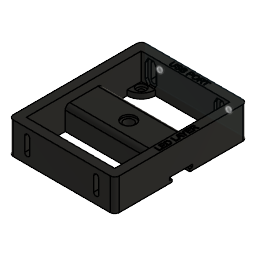
LED-LAYER (Autodesk Fusion 360 design; units mm, degrees)
part number: 2026-05-15-16-15-28-168
Autodesk Fusion 360 part; units mm, degrees
note: some values were not read from the file. Chosen so that the rebuilt part matches the saved one: which face or edge a step refers to; a direction; the layout of a text. Set by a fixed rule: which sketch regions a step uses.
sketch "Sketch1" plane through (0, 0, 0) normal (0, 0, 1) x (1, 0, 0)
  line L0 (2.5, 0) -> (57.5, 0)
  line L1 (60, 2.5) -> (60, 72.5)
  line L2 (57.5, 75) -> (2.5, 75)
  line L3 (0, 72.5) -> (0, 2.5)
  arc A0 (0, 2.5) -> (2.5, 0) centre (2.5, 2.5) ccw
  arc A1 (57.5, 0) -> (60, 2.5) centre (57.5, 2.5) ccw
  arc A2 (60, 72.5) -> (57.5, 75) centre (57.5, 72.5) ccw
  arc A3 (2.5, 75) -> (0, 72.5) centre (2.5, 72.5) ccw
  point P0 (60, 0)
  point P1 (0, 75)
  dimension "d1" = 60
  dimension "d2" = 75
  dimension "d3" = 2.5
  constraint horizontal L0
  constraint vertical L1
  constraint horizontal L2
  constraint vertical L3
  constraint coincident origin L0
  constraint coincident origin L3
  constraint tangent L0 A0
  constraint tangent L3 A0
  constraint coincident P0 L0
  constraint coincident P0 L1
  constraint tangent L0 A1
  constraint tangent L1 A1
  constraint equal A0 A1
  constraint tangent L1 A2
  constraint tangent L2 A2
  constraint equal A0 A2
  constraint coincident P1 L2
  constraint coincident P1 L3
  constraint tangent L2 A3
  constraint tangent L3 A3
  constraint equal A0 A3
  measures "d1" distance of origin P0
  measures "d2" distance of origin P1
  measures "d3" radius of A0
extrude "Extrude1" add sketch "Sketch1" along normal blind 6
sketch "Sketch2" plane through (60, 0, 0) normal (1, 0, 0) x (0, 1, 0)
  line L0 (2.5, 0) -> (72.5, 0)
  line L1 (72.5, 0) -> (72.5, 6)
  line L2 (72.5, 6) -> (2.5, 6)
  line L3 (2.5, 6) -> (2.5, 0)
  line L4 (32.5, 0) -> (42.5, 0)
  line L5 (42.5, 0) -> (42.5, 3)
  line L6 (42.5, 3) -> (32.5, 3)
  line L7 (32.5, 3) -> (32.5, 0)
  line L8 (0, 0) -> (0, 6)
  dimension "d6" = 10
  dimension "d7" = 3
  dimension "d8" = 32.5
  constraint horizontal L4
  constraint vertical L5
  constraint horizontal L6
  constraint vertical L7
  constraint coincident L0 L4.start
  measures "d6" distance of L4.start L4.end
  measures "d7" distance of L4.start L6.end
  measures "d8" distance of L7 L8
extrude "Extrude2" cut sketch "Sketch2" against normal blind 60 contours L0 L4 L5 L6 L7
sketch "Sketch3" plane through (60, 0, 0) normal (1, 0, 0) x (0, 1, 0)
  line L0 (42.5, 3) -> (42.5, 0)
  line L1 (42.5, 0) -> (72.5, 0)
  line L2 (72.5, 0) -> (72.5, 6)
  line L3 (72.5, 6) -> (2.5, 6)
  line L4 (2.5, 6) -> (2.5, 0)
  line L5 (2.5, 0) -> (32.5, 0)
  line L6 (32.5, 0) -> (32.5, 3)
  line L7 (32.5, 3) -> (42.5, 3)
  line L8 (30, 5) -> (45, 5)
  line L9 (45, 5) -> (45, 3)
  line L10 (45, 3) -> (30, 3)
  line L11 (30, 3) -> (30, 5)
  dimension "d11" = 2.5
  constraint horizontal L8
  constraint vertical L9
  constraint horizontal L10
  constraint vertical L11
  measures "d11" distance of L6 L11
extrude "Extrude3" cut sketch "Sketch3" along normal blind 60 contours L7 L8 L9 L10 L11
sketch "Sketch4" plane through (0, 0, 6) normal (0, 0, 1) x (-1, 0, 0)
  arc A0 (-2.5, -75) -> (0, -72.5) centre (-2.5, -72.5) ccw
  line L0 (0, -72.5) -> (0, -2.5)
  arc A1 (0, -2.5) -> (-2.5, 0) centre (-2.5, -2.5) ccw
  line L1 (-2.5, 0) -> (-57.5, 0)
  arc A2 (-57.5, 0) -> (-60, -2.5) centre (-57.5, -2.5) ccw
  line L2 (-60, -2.5) -> (-60, -72.5)
  arc A3 (-60, -72.5) -> (-57.5, -75) centre (-57.5, -72.5) ccw
  line L3 (-57.5, -75) -> (-2.5, -75)
  circle A4 centre (-29.575, -37.5) radius 2.6
  line L4 (-5, -5) -> (-55, -5)
  line L5 (-55, -5) -> (-55, -70)
  line L6 (-55, -70) -> (-5, -70)
  line L7 (-5, -70) -> (-5, -5)
  dimension "d14" = 5.2
  dimension "d15" = 37.5
  dimension "d16" = 30.425
  constraint horizontal L4
  constraint vertical L5
  constraint horizontal L6
  constraint vertical L7
  measures "d14" diameter of A4
  measures "d15" distance of L1 A4.centre
  measures "d16" distance of L2 A4.centre
extrude "Extrude4" add sketch "Sketch4" along normal blind 7 contours A0 L0 A1 L1 A2 L2 A3 L3 | L4 L5 L6 L7
extrude "Extrude5" cut 1 faces at (30.432, 36.8771, 6) along direction (0, 0, -1) blind 1
extrude "Extrude6" cut sketch "Sketch4" against normal blind 1 contours L4 L5 L6 L7
sketch "Sketch5" plane through (0, 0, 13) normal (0, 0, 1) x (-1, 0, 0)
  circle A0 centre (-29.575, -37.5) radius 2.6
  line L0 (-57.5, -75) -> (-2.5, -75)
  arc A1 (-2.5, -75) -> (0, -72.5) centre (-2.5, -72.5) ccw
  line L1 (0, -72.5) -> (0, -2.5)
  arc A2 (0, -2.5) -> (-2.5, 0) centre (-2.5, -2.5) ccw
  line L2 (-2.5, 0) -> (-57.5, 0)
  arc A3 (-57.5, 0) -> (-60, -2.5) centre (-57.5, -2.5) ccw
  line L3 (-60, -2.5) -> (-60, -72.5)
  arc A4 (-60, -72.5) -> (-57.5, -75) centre (-57.5, -72.5) ccw
  line L4 (-5, -5) -> (-55, -5)
  line L5 (-55, -5) -> (-55, -70)
  line L6 (-55, -70) -> (-5, -70)
  line L7 (-5, -70) -> (-5, -5)
  circle A5 centre (-29.575, -37.5) radius 5
  line L8 (-5, -30) -> (-55, -30)
  line L9 (-55, -30) -> (-55, -45)
  line L10 (-55, -45) -> (-5, -45)
  line L11 (-5, -45) -> (-5, -30)
  dimension "d23" = 10
  constraint horizontal L4
  constraint vertical L5
  constraint horizontal L6
  constraint vertical L7
  constraint concentric A0 A5
  constraint horizontal L8
  constraint vertical L9
  constraint horizontal L10
  constraint vertical L11
  constraint coincident L5 L9.end
  constraint coincident L7 L8.start
  measures "d23" diameter of A5
extrude "Extrude7" cut sketch "Sketch5" against normal blind 7 contours L4 L5 L7 L8 | L5 L6 L7 L10
sketch "Sketch6" plane through (0, 0, 13) normal (0, 0, 1) x (-1, 0, 0)
  line L0 (-5, -27) -> (-55, -27)
  line L1 (-55, -27) -> (-55, -5)
  line L2 (-55, -5) -> (-5, -5)
  line L3 (-5, -5) -> (-5, -27)
  line L4 (-5, -48) -> (-55, -48)
  line L5 (-55, -48) -> (-55, -70)
  line L6 (-55, -70) -> (-5, -70)
  line L7 (-5, -70) -> (-5, -48)
  constraint horizontal L0
  constraint vertical L1
  constraint horizontal L2
  constraint vertical L3
  constraint horizontal L4
  constraint vertical L5
  constraint horizontal L6
  constraint vertical L7
extrude "Extrude9" cut sketch "Sketch6" against normal blind 20
sketch "Sketch7" plane through (0, 0, 13) normal (0, 0, 1) x (-1, 0, 0)
  line L0 (-5, -45) -> (-5, -70)
  line L1 (-5, -70) -> (-55, -70)
  line L2 (-55, -70) -> (-55, -45)
  line L3 (-55, -45) -> (-5, -45)
  line L4 (-55, -30) -> (-55, -5)
  line L5 (-55, -5) -> (-5, -5)
  line L6 (-5, -5) -> (-5, -30)
  line L7 (-5, -30) -> (-55, -30)
  circle A0 centre (-29.575, -37.5) radius 2.6
  line L8 (-57.5, -75) -> (-2.5, -75)
  arc A1 (-2.5, -75) -> (0, -72.5) centre (-2.5, -72.5) ccw
  line L9 (0, -72.5) -> (0, -2.5)
  arc A2 (0, -2.5) -> (-2.5, 0) centre (-2.5, -2.5) ccw
  line L10 (-2.5, 0) -> (-57.5, 0)
  arc A3 (-57.5, 0) -> (-60, -2.5) centre (-57.5, -2.5) ccw
  line L11 (-60, -2.5) -> (-60, -72.5)
  arc A4 (-60, -72.5) -> (-57.5, -75) centre (-57.5, -72.5) ccw
  line L12 (-5, -30) -> (-5, -45)
  line L13 (-55, -45) -> (-55, -30)
  constraint coincident L6.end L7.start
  constraint coincident L0.start L3.end
  constraint coincident L2.end L3.start
  constraint coincident L4.start L7.end
extrude "Extrude10" add sketch "Sketch7" along normal blind 5 contours L8 A1 L9 A2 L10 A3 L11 A4
sketch "Sketch8" plane through (0, 5, 0) normal (0, 1, 0) x (-1, 0, 0)
  line L0 (-55, 13) -> (-55, 0)
  line L1 (-55, 0) -> (-5, 0)
  line L2 (-5, 0) -> (-5, 18)
  line L3 (-5, 18) -> (-55, 18)
  line L4 (-55, 18) -> (-55, 13)
  line L5 (-5, 0) -> (-13, 0)
  line L6 (-13, 0) -> (-13, 3)
  line L7 (-13, 3) -> (-5, 3)
  line L8 (-5, 3) -> (-5, 0)
  line L9 (-55, 0) -> (-47, 0)
  line L10 (-47, 0) -> (-47, 3)
  line L11 (-47, 3) -> (-55, 3)
  line L12 (-55, 3) -> (-55, 0)
  dimension "d32" = 8
  dimension "d33" = 3
  dimension "d34" = 8
  dimension "d35" = 3
  constraint horizontal L5
  constraint vertical L6
  constraint horizontal L7
  constraint vertical L8
  constraint coincident L1.end L2.start
  constraint horizontal L9
  constraint vertical L10
  constraint horizontal L11
  constraint vertical L12
  constraint coincident L0.end L1.start
  measures "d32" distance of L1.end L5.end
  measures "d33" distance of L1.end L7.end
  measures "d34" distance of L0.end L9.end
  measures "d35" distance of L0.end L11.end
extrude "Extrude11" add sketch "Sketch8" along normal blind 8 contours L0 L1 L9 L10 L11 L12 | L1 L2 L5 L6 L7 L8
sketch "Sketch9" plane through (0, 70, 0) normal (0, -1, 0) x (1, 0, 0)
  line L0 (5, 18) -> (5, 0)
  line L1 (5, 0) -> (55, 0)
  line L2 (55, 0) -> (55, 13)
  line L3 (55, 13) -> (55, 18)
  line L4 (55, 18) -> (5, 18)
  line L5 (5, 0) -> (13, 0)
  line L6 (13, 0) -> (13, 3)
  line L7 (13, 3) -> (5, 3)
  line L8 (5, 3) -> (5, 0)
  line L9 (55, 0) -> (47, 0)
  line L10 (47, 0) -> (47, 3)
  line L11 (47, 3) -> (55, 3)
  line L12 (55, 3) -> (55, 0)
  dimension "d38" = 8
  dimension "d39" = 3
  dimension "d40" = 8
  dimension "d41" = 3
  constraint horizontal L5
  constraint vertical L6
  constraint horizontal L7
  constraint vertical L8
  constraint coincident L0.end L1.start
  constraint horizontal L9
  constraint vertical L10
  constraint horizontal L11
  constraint vertical L12
  constraint coincident L1.end L2.start
  measures "d38" distance of L0.end L5.end
  measures "d39" distance of L0.end L7.end
  measures "d40" distance of L1.end L9.end
  measures "d41" distance of L1.end L11.end
extrude "Extrude12" add sketch "Sketch9" along normal blind 8 contours L0 L1 L5 L6 L7 L8 | L1 L2 L9 L10 L11 L12
extrude "Extrude13" add 2 faces at (21.6667, 41, 5) (21.6667, 41, 5) along direction (0, 0, 1) blind 8
sketch "Sketch10" plane through (0, 0, 3) normal (0, 0, 1) x (-1, 0, 0)
  line L0 (-55, -70) -> (-47, -70)
  line L1 (-47, -70) -> (-47, -62)
  line L2 (-47, -62) -> (-55, -62)
  line L3 (-55, -62) -> (-55, -70)
  circle A0 centre (-52, -67) radius 1.4
  line L4 (-55, -5) -> (-55, -70)
  line L5 (-55, -70) -> (-5, -70)
  circle A1 centre (-52, -8) radius 1.4
  line L6 (-5, -5) -> (-55, -5)
  circle A2 centre (-8, -67) radius 1.4
  line L7 (-5, -70) -> (-5, -5)
  circle A3 centre (-8, -8) radius 1.4
  dimension "d46" = 2.8
  dimension "d47" = 3
  dimension "d48" = 3
  dimension "d49" = 2.8
  dimension "d50" = 3
  dimension "d51" = 3
  dimension "d52" = 2.8
  dimension "d53" = 3
  dimension "d54" = 3
  dimension "d55" = 2.8
  dimension "d56" = 3
  dimension "d57" = 3
  measures "d46" diameter of A0
  measures "d47" distance of A0.centre L4
  measures "d48" distance of A0.centre L5
  measures "d49" diameter of A1
  measures "d50" distance of L4 A1.centre
  measures "d51" distance of A1.centre L6
  measures "d52" diameter of A2
  measures "d53" distance of L5 A2.centre
  measures "d54" distance of A2.centre L7
  measures "d55" diameter of A3
  measures "d56" distance of L6 A3.centre
  measures "d57" distance of L7 A3.centre
extrude "Extrude14" cut sketch "Sketch10" against normal blind 3 contours A0 | A1 | A2 | A3
sketch "Sketch11" plane through (0, 0, 3) normal (0, 0, 1) x (-1, 0, 0)
  circle A0 centre (-52, -67) radius 1.4
  line L0 (-55, -70) -> (-47, -70)
  line L1 (-47, -70) -> (-47, -62)
  line L2 (-47, -62) -> (-55, -62)
  line L3 (-55, -62) -> (-55, -70)
  arc A1 (-47, -70) -> (-55, -62) centre (-55, -70) ccw
  arc A2 (-5, -62) -> (-13, -70) centre (-5, -70) ccw
  arc A3 (-13, -5) -> (-5, -13) centre (-5, -5) ccw
  arc A4 (-55, -13) -> (-47, -5) centre (-55, -5) ccw
  line L4 (-13, -70) -> (-13, -62)
  line L5 (-13, -62) -> (-5, -62)
  line L6 (-5, -13) -> (-13, -13)
  line L7 (-13, -13) -> (-13, -5)
  line L8 (-55, -13) -> (-47, -13)
  line L9 (-47, -13) -> (-47, -5)
  constraint coincident L0 L1.start
  constraint coincident L2.end L3.start
  constraint coincident L0.start L3.end
  constraint tangent A2 L4
  constraint vertical L4
  constraint tangent A2 L5
  constraint tangent A3 L6
  constraint parallel L5 L6
  constraint tangent A3 L7
  constraint tangent A4 L8
  constraint perpendicular L7 L8
  constraint tangent A4 L9
extrude "Extrude15" cut sketch "Sketch11" against normal blind 3 contours L1 L2 A1 | A2 L4 L5 | A3 L6 L7 | A4 L8 L9
sketch "Sketch12" plane through (0, 0, 18) normal (0, 0, 1) x (-1, 0, 0)
  line L0 (-55, -70) -> (-55, -45)
  line L1 (-55, -45) -> (-55, -30)
  line L2 (-55, -30) -> (-55, -5)
  line L3 (-55, -5) -> (-5, -5)
  line L4 (-5, -5) -> (-5, -70)
  line L5 (-5, -70) -> (-55, -70)
  arc A0 (-60, -72.5) -> (-57.5, -75) centre (-57.5, -72.5) ccw
  line L6 (-57.5, -75) -> (-2.5, -75)
  arc A1 (-2.5, -75) -> (0, -72.5) centre (-2.5, -72.5) ccw
  line L7 (0, -72.5) -> (0, -2.5)
  arc A2 (0, -2.5) -> (-2.5, 0) centre (-2.5, -2.5) ccw
  line L8 (-2.5, 0) -> (-57.5, 0)
  arc A3 (-57.5, 0) -> (-60, -2.5) centre (-57.5, -2.5) ccw
  line L9 (-60, -2.5) -> (-60, -72.5)
  line L10 (-13, -70) -> (-47, -70) construction
  line L11 (-47, -70) -> (-47, -75) construction
  line L12 (-47, -75) -> (-13, -75) construction
  line L13 (-13, -75) -> (-13, -70) construction
  line L14 (-60, -13) -> (-60, -62) construction
  line L15 (-60, -62) -> (-55, -62) construction
  line L16 (-55, -62) -> (-55, -13) construction
  line L17 (-55, -13) -> (-60, -13) construction
  dimension "d62" = 3
  dimension "d64" = 3
  text T0 "USB PORT" font "Arial" height 3 align centre middle in box 34 x 5 at (-13, -70) x (-1, 0) y (0, -1) spacing 1 kerned
  text T1 "LED LAYER" font "Arial" height 3 align centre middle in box 49 x 5 at (-60, -13) x (0, -1) y (1, 0) spacing 1 kerned
  constraint coincident L6
  constraint coincident L5
  constraint coincident L0
  constraint coincident L9
extrude "Extrude16" cut sketch "Sketch12" against normal blind 2 text T1 T0
fillet "Fillet1" radius 2.5 2 edges at (30, 48, 13) (30, 27, 13)
sketch "Sketch13" plane through (0, 0, 0) normal (0, -1, 0) x (1, 0, 0)
  line L0 (2.5, 0) -> (57.5, 0)
  line L1 (57.5, 0) -> (57.5, 18)
  line L2 (57.5, 18) -> (2.5, 18)
  line L3 (2.5, 18) -> (2.5, 0)
  circle A0 centre (10.5, 9) radius 1.4
  circle A1 centre (49.5, 9) radius 1.4
  dimension "d70" = 2.8
  dimension "d71" = 9
  dimension "d72" = 8
  dimension "d73" = 2.8
  dimension "d74" = 8
  dimension "d75" = 9
  measures "d70" diameter of A0
  measures "d71" distance of L2 A0.centre
  measures "d72" distance of L3 A0.centre
  measures "d73" diameter of A1
  measures "d74" distance of L1 A1.centre
  measures "d75" distance of L2 A1.centre
extrude "Extrude17" cut sketch "Sketch13" against normal blind 6 contours A0 | A1
sketch "Sketch14" plane through (0, 75, 0) normal (0, 1, 0) x (-1, 0, 0)
  line L0 (-57.5, 0) -> (-2.5, 0)
  line L1 (-2.5, 0) -> (-2.5, 18)
  line L2 (-2.5, 18) -> (-57.5, 18)
  line L3 (-57.5, 18) -> (-57.5, 0)
  circle A0 centre (-49.5, 9) radius 1.4
  circle A1 centre (-10.5, 9) radius 1.4
  dimension "d78" = 2.8
  dimension "d79" = 9
  dimension "d80" = 8
  dimension "d81" = 2.8
  dimension "d82" = 9
  dimension "d83" = 8
  measures "d78" diameter of A0
  measures "d79" distance of L0 A0.centre
  measures "d80" distance of L3 A0.centre
  measures "d81" diameter of A1
  measures "d82" distance of L0 A1.centre
  measures "d83" distance of L1 A1.centre
extrude "Extrude18" cut sketch "Sketch14" against normal blind 6 contours A0 | A1
sketch "Sketch15" plane through (0, 0, 5) normal (0, 0, -1) x (1, 0, 0)
  line L0 (5, -45) -> (5, -30)
  line L1 (5, -30) -> (0, -30)
  line L2 (0, -30) -> (0, -45)
  line L3 (0, -45) -> (5, -45)
  line L4 (0, -45) -> (5, -45)
  line L5 (5, -45) -> (5, -30)
  line L6 (5, -30) -> (0, -30)
  line L7 (0, -30) -> (0, -45)
  constraint horizontal L4
  constraint vertical L5
  constraint horizontal L6
  constraint vertical L7
  constraint coincident L0.end L1.start
  constraint coincident L2.end L3.start
extrude "Extrude19" add sketch "Sketch15" along normal blind 5
sketch "Sketch16" plane through (0, 0, 13) normal (0, 0, 1) x (-1, 0, 0)
  line L0 (-5, -29.5) -> (-55, -29.5)
  line L1 (-55, -29.5) -> (-55, -30)
  line L2 (-55, -30) -> (-55, -45)
  line L3 (-55, -45) -> (-55, -45.5)
  line L4 (-55, -45.5) -> (-5, -45.5)
  line L5 (-5, -45.5) -> (-5, -29.5)
  circle A0 centre (-30.425, -37.5) radius 4
  line L6 (0, -72.5) -> (0, -2.5)
  circle A1 centre (-30.425, -37.5) radius 2.7
  dimension "d88" = 8
  dimension "d159" = 30.425
  dimension "d160" = 5.4
  constraint concentric A0 A1
  measures "d88" diameter of A0
  measures "d159" distance of A0.centre L6
  measures "d160" diameter of A1
extrude "Extrude20" cut sketch "Sketch16" against normal blind 1 contours A0 | A1
sketch "Sketch17" plane through (0, 0, 3) normal (0, 0, 1) x (-1, 0, 0)
  arc A0 (-13, -5) -> (-5, -13) centre (-5, -5) ccw
  line L0 (-5, -13) -> (-5, -5)
  line L1 (-5, -5) -> (-13, -5)
  circle A1 centre (-8, -8) radius 1.4
  circle A2 centre (-8, -8) radius 2.75
  circle A3 centre (-52, -8) radius 2.75
  circle A4 centre (-8, -67) radius 2.75
  circle A5 centre (-52, -67) radius 2.75
  dimension "d91" = 5.5
  dimension "d92" = 5.5
  dimension "d93" = 5.5
  dimension "d94" = 5.5
  constraint concentric A1 A2
  measures "d91" diameter of A2
  measures "d92" diameter of A3
  measures "d93" diameter of A4
  measures "d94" diameter of A5
extrude "Extrude21" cut sketch "Sketch17" against normal blind 1.5 contours A2 | A3 | A4 | A5
sketch "Sketch18" plane through (0, 70, 0) normal (0, -1, 0) x (1, 0, 0)
  circle A0 centre (10.5, 9) radius 1.4
  circle A1 centre (49.5, 9) radius 1.4
  line L0 (13, 3) -> (13, 0)
  line L1 (13, 0) -> (47, 0)
  line L2 (47, 0) -> (47, 3)
  line L3 (47, 3) -> (55, 3)
  line L4 (55, 3) -> (55, 13)
  line L5 (55, 13) -> (55, 18)
  line L6 (55, 18) -> (5, 18)
  line L7 (5, 18) -> (5, 3)
  line L8 (5, 3) -> (13, 3)
  line L9 (13.6336, 8.2037) -> (12.7564, 11.3156)
  line L10 (12.7564, 11.3156) -> (9.6229, 12.1119)
  line L11 (9.6229, 12.1119) -> (7.3664, 9.7963)
  line L12 (7.3664, 9.7963) -> (8.2436, 6.6844)
  line L13 (8.2436, 6.6844) -> (11.3771, 5.8881)
  line L14 (11.3771, 5.8881) -> (13.6336, 8.2037)
  line L15 (52.301, 7.3852) -> (52.299, 10.6183)
  line L16 (52.299, 10.6183) -> (49.498, 12.2332)
  line L17 (49.498, 12.2332) -> (46.699, 10.6148)
  line L18 (46.699, 10.6148) -> (46.701, 7.3817)
  line L19 (46.701, 7.3817) -> (49.502, 5.7668)
  line L20 (49.502, 5.7668) -> (52.301, 7.3852)
  point P0 (10.5, 9)
  point P1 (49.5, 9)
  dimension "d97" = 2.8
  dimension "d98" = 2.8
  constraint coincident P0 A0.centre
  constraint coincident P1 A1.centre
  measures "d97" distance of P0 L14
  measures "d98" distance of P1 L20
sketch "Sketch19" plane through (0, 5, 0) normal (0, 1, 0) x (-1, 0, 0)
  circle A0 centre (-10.5, 9) radius 1.4
  circle A1 centre (-49.5, 9) radius 1.4
  line L0 (-47, 3) -> (-47, 0)
  line L1 (-47, 0) -> (-13, 0)
  line L2 (-13, 0) -> (-13, 3)
  line L3 (-13, 3) -> (-5, 3)
  line L4 (-5, 3) -> (-5, 18)
  line L5 (-5, 18) -> (-55, 18)
  line L6 (-55, 18) -> (-55, 13)
  line L7 (-55, 13) -> (-55, 3)
  line L8 (-55, 3) -> (-47, 3)
  line L9 (-46.5267, 7.7299) -> (-46.9135, 10.9399)
  line L10 (-46.9135, 10.9399) -> (-49.8867, 12.2099)
  line L11 (-49.8867, 12.2099) -> (-52.4733, 10.2701)
  line L12 (-52.4733, 10.2701) -> (-52.0865, 7.0601)
  line L13 (-52.0865, 7.0601) -> (-49.1133, 5.7901)
  line L14 (-49.1133, 5.7901) -> (-46.5267, 7.7299)
  line L15 (-10.3689, 5.7695) -> (-7.6368, 7.4983)
  line L16 (-7.6368, 7.4983) -> (-7.7679, 10.7288)
  line L17 (-7.7679, 10.7288) -> (-10.6311, 12.2305)
  line L18 (-10.6311, 12.2305) -> (-13.3632, 10.5017)
  line L19 (-13.3632, 10.5017) -> (-13.2321, 7.2712)
  line L20 (-13.2321, 7.2712) -> (-10.3689, 5.7695)
  point P0 (-49.5, 9)
  point P1 (-10.5, 9)
  dimension "d101" = 2.8
  dimension "d102" = 2.8
  constraint coincident P0 A1.centre
  constraint coincident A0.centre P1
  measures "d101" distance of P0 L14
  measures "d102" distance of P1 L20
sketch "Sketch20" plane through (0, 0, 0) normal (0, 1, 0) x (1, 0, 0)
  line L0 (9.1, -9) -> (11.9, -9)
  line L1 (11.9, -9) -> (11.9, -13.6)
  line L2 (9.1, -13.6) -> (9.1, -9)
  arc A0 (9.1, -13.6) -> (10.5, -15) centre (10.5, -13.6) ccw
  arc A1 (10.5, -15) -> (11.9, -13.6) centre (10.5, -13.6) ccw
  line L3 (9.1, -9) -> (11.9, -9)
  line L4 (48.1, -9) -> (50.9, -9)
  line L5 (50.9, -9) -> (50.9, -13.6)
  line L6 (48.1, -13.6) -> (48.1, -9)
  line L7 (48.1, -9) -> (50.9, -9)
  arc A2 (48.1, -13.6) -> (49.5, -15) centre (49.5, -13.6) ccw
  arc A3 (49.5, -15) -> (50.9, -13.6) centre (49.5, -13.6) ccw
  line L8 (48.1, -9) -> (50.9, -9)
  line L9 (50.9, -9) -> (50.9, -5.4)
  line L10 (48.1, -5.4) -> (48.1, -9)
  arc A4 (49.5, -4) -> (48.1, -5.4) centre (49.5, -5.4) ccw
  arc A5 (50.9, -5.4) -> (49.5, -4) centre (49.5, -5.4) ccw
  line L11 (9.1, -9) -> (11.9, -9)
  line L12 (11.9, -9) -> (11.9, -5.4)
  line L13 (9.1, -5.4) -> (9.1, -9)
  arc A6 (10.5, -4) -> (9.1, -5.4) centre (10.5, -5.4) ccw
  arc A7 (11.9, -5.4) -> (10.5, -4) centre (10.5, -5.4) ccw
  point P0 (9.1, -15)
  point P1 (48.1, -15)
  point P2 (48.1, -4)
  point P3 (9.1, -4)
  dimension "d105" = 2.8
  dimension "d106" = 6
  dimension "d107" = 1.4
  dimension "d108" = 1.4
  dimension "d111" = 2.8
  dimension "d112" = 6
  dimension "d115" = 1.4
  dimension "d118" = 5
  dimension "d119" = 1.4
  dimension "d120" = 5
  dimension "d121" = 1.4
  constraint horizontal L0
  constraint vertical L1
  constraint vertical L2
  constraint coincident P0 L2
  constraint tangent L2 A0
  constraint tangent L1 A1
  constraint coincident A0.end A1.start
  constraint horizontal L3
  constraint horizontal L4
  constraint vertical L5
  constraint vertical L6
  constraint horizontal L7
  constraint coincident P1 L6
  constraint tangent L6 A2
  constraint tangent L5 A3
  constraint equal A2 A3
  constraint coincident A2.end A3.start
  constraint horizontal L8
  constraint vertical L9
  constraint vertical L10
  constraint coincident P2 L10
  constraint tangent L10 A4
  constraint tangent L9 A5
  constraint equal A4 A5
  constraint coincident A4.start A5.end
  constraint horizontal L11
  constraint vertical L12
  constraint vertical L13
  constraint coincident P3 L13
  constraint tangent L13 A6
  constraint tangent L12 A7
  constraint equal A6 A7
  constraint coincident A6.start A7.end
  measures "d105" distance of L0.start L0.end
  measures "d106" distance of L0.start P0
  measures "d107" radius of A0
  measures "d108" radius of A1
  measures "d111" distance of L4.start L4.end
  measures "d112" distance of L4.start P1
  measures "d115" radius of A2
  measures "d118" distance of L4.start P2
  measures "d119" radius of A4
  measures "d120" distance of L0.start P3
  measures "d121" radius of A6
extrude "Extrude25" cut sketch "Sketch20" along normal blind 6
sketch "Sketch21" plane through (0, 5, 0) normal (0, 1, 0) x (-1, 0, 0)
  line L0 (-11.9, 5.4) -> (-11.9, 13.6)
  arc A0 (-9.1, 13.6) -> (-11.9, 13.6) centre (-10.5, 13.6) ccw
  line L1 (-9.1, 13.6) -> (-9.1, 5.4)
  arc A1 (-11.9, 5.4) -> (-9.1, 5.4) centre (-10.5, 5.4) ccw
  line L2 (-50.9, 5.4) -> (-50.9, 13.6)
  arc A2 (-48.1, 13.6) -> (-50.9, 13.6) centre (-49.5, 13.6) ccw
  line L3 (-48.1, 13.6) -> (-48.1, 5.4)
  arc A3 (-50.9, 5.4) -> (-48.1, 5.4) centre (-49.5, 5.4) ccw
  line L4 (-47, 3) -> (-47, 0)
  line L5 (-47, 0) -> (-13, 0)
  line L6 (-13, 0) -> (-13, 3)
  line L7 (-13, 3) -> (-5, 3)
  line L8 (-5, 3) -> (-5, 18)
  line L9 (-5, 18) -> (-55, 18)
  line L10 (-55, 18) -> (-55, 13)
  line L11 (-55, 13) -> (-55, 3)
  line L12 (-55, 3) -> (-47, 3)
  line L13 (-47.8834, 2.6) -> (-46.2668, 5.4)
  line L14 (-46.2668, 5.4) -> (-47.8834, 8.2)
  line L15 (-47.8834, 8.2) -> (-51.1166, 8.2)
  line L16 (-51.1166, 8.2) -> (-52.7332, 5.4)
  line L17 (-52.7332, 5.4) -> (-51.1166, 2.6)
  line L18 (-51.1166, 2.6) -> (-47.8834, 2.6)
  line L19 (-47.8834, 10.8) -> (-46.2668, 13.6)
  line L20 (-46.2668, 13.6) -> (-47.8834, 16.4)
  line L21 (-47.8834, 16.4) -> (-51.1166, 16.4)
  line L22 (-51.1166, 16.4) -> (-52.7332, 13.6)
  line L23 (-52.7332, 13.6) -> (-51.1166, 10.8)
  line L24 (-51.1166, 10.8) -> (-47.8834, 10.8)
  line L25 (-46.2668, 13.6) -> (-46.2668, 5.4)
  line L26 (-52.7332, 5.4) -> (-52.7332, 13.6)
  line L27 (-8.8834, 10.8) -> (-7.2668, 13.6)
  line L28 (-7.2668, 13.6) -> (-8.8834, 16.4)
  line L29 (-8.8834, 16.4) -> (-12.1166, 16.4)
  line L30 (-12.1166, 16.4) -> (-13.7332, 13.6)
  line L31 (-13.7332, 13.6) -> (-12.1166, 10.8)
  line L32 (-12.1166, 10.8) -> (-8.8834, 10.8)
  line L33 (-8.8834, 2.6) -> (-7.2668, 5.4)
  line L34 (-7.2668, 5.4) -> (-8.8834, 8.2)
  line L35 (-8.8834, 8.2) -> (-12.1166, 8.2)
  line L36 (-12.1166, 8.2) -> (-13.7332, 5.4)
  line L37 (-13.7332, 5.4) -> (-12.1166, 2.6)
  line L38 (-12.1166, 2.6) -> (-8.8834, 2.6)
  line L39 (-13.7332, 13.6) -> (-13.7332, 5.4)
  line L40 (-7.2668, 5.4) -> (-7.2668, 13.6)
  point P0 (-49.5, 5.4)
  point P1 (-49.5, 13.6)
  point P2 (-10.5, 13.6)
  point P3 (-10.5, 5.4)
  dimension "d124" = 2.8
  dimension "d125" = 2.8
  dimension "d126" = 2.8
  dimension "d127" = 2.8
  constraint coincident P0 A3.centre
  constraint coincident P1 A2.centre
  constraint vertical L25
  constraint coincident P2 A0.centre
  constraint coincident P3 A1.centre
  constraint vertical L39
  measures "d124" distance of P0 L18
  measures "d125" distance of P1 L24
  measures "d126" distance of P2 L32
  measures "d127" distance of P3 L38
extrude "Extrude26" cut sketch "Sketch21" against normal blind 1.5 contours L0 L1 A1 L7 L33 L34 L35 L36 L37 | L0 L1 A1 L35 | L0 L31 L32 L35 L36 L39 | L0 L1 L32 L35 | L0 A0 L1 L27 L28 L29 L30 L31 L32 | L0 A0 L1 L32 | L1 L27 L32 L34 L35 L40 | L2 L3 A3 L12 L13 L14 L15 L16 L17 | L3 L14 L15 L19 L24 L25 | L2 L15 L16 L23 L24 L26 | L2 A2 L3 L19 L20 L21 L22 L23 L24 | L2 L3 L15 L24 | L2 L3 A3 L15 | L2 A2 L3 L24
sketch "Sketch22" plane through (0, 70, 0) normal (0, -1, 0) x (1, 0, 0)
  circle A0 centre (10.5, 9) radius 1.4
  circle A1 centre (49.5, 9) radius 1.4
  line L0 (13, 3) -> (13, 0)
  line L1 (13, 0) -> (47, 0)
  line L2 (47, 0) -> (47, 3)
  line L3 (47, 3) -> (55, 3)
  line L4 (55, 3) -> (55, 13)
  line L5 (55, 13) -> (55, 18)
  line L6 (55, 18) -> (5, 18)
  line L7 (5, 18) -> (5, 3)
  line L8 (5, 3) -> (13, 3)
  line L9 (9.1, 9) -> (11.9, 9)
  line L10 (11.9, 9) -> (11.9, 13.6)
  line L11 (9.1, 13.6) -> (9.1, 9)
  line L12 (9.1, 9) -> (11.9, 9)
  line L13 (11.9, 9) -> (11.9, 5.4)
  line L14 (9.1, 5.4) -> (9.1, 9)
  line L15 (48.1, 9) -> (50.9, 9)
  line L16 (50.9, 9) -> (50.9, 13.6)
  line L17 (48.1, 13.6) -> (48.1, 9)
  line L18 (48.1, 9) -> (50.9, 9)
  line L19 (50.9, 9) -> (50.9, 5.4)
  line L20 (48.1, 5.4) -> (48.1, 9)
  arc A2 (10.5, 15) -> (9.1, 13.6) centre (10.5, 13.6) ccw
  arc A3 (11.9, 13.6) -> (10.5, 15) centre (10.5, 13.6) ccw
  arc A4 (9.1, 5.4) -> (10.5, 4) centre (10.5, 5.4) ccw
  arc A5 (10.5, 4) -> (11.9, 5.4) centre (10.5, 5.4) ccw
  arc A6 (49.5, 15) -> (48.1, 13.6) centre (49.5, 13.6) ccw
  arc A7 (50.9, 13.6) -> (49.5, 15) centre (49.5, 13.6) ccw
  arc A8 (48.1, 5.4) -> (49.5, 4) centre (49.5, 5.4) ccw
  arc A9 (49.5, 4) -> (50.9, 5.4) centre (49.5, 5.4) ccw
  point P0 (9.1, 15)
  point P1 (9.1, 4)
  point P2 (48.1, 15)
  point P3 (48.1, 4)
  dimension "d130" = 2.8
  dimension "d131" = 6
  dimension "d132" = 5
  dimension "d133" = 2.8
  dimension "d134" = 6
  dimension "d135" = 5
  dimension "d136" = 1.4
  dimension "d137" = 1.4
  dimension "d138" = 1.4
  dimension "d139" = 1.4
  constraint horizontal L9
  constraint vertical L10
  constraint vertical L11
  constraint coincident A0 L9.start
  constraint horizontal L12
  constraint vertical L13
  constraint vertical L14
  constraint horizontal L15
  constraint vertical L16
  constraint vertical L17
  constraint coincident A1 L15.start
  constraint horizontal L18
  constraint vertical L19
  constraint vertical L20
  constraint coincident P0 L11
  constraint tangent L11 A2
  constraint tangent L10 A3
  constraint equal A2 A3
  constraint coincident A2.start A3.end
  constraint coincident P1 L14
  constraint tangent L14 A4
  constraint tangent L13 A5
  constraint equal A4 A5
  constraint coincident A4.end A5.start
  constraint coincident P2 L17
  constraint tangent L17 A6
  constraint tangent L16 A7
  constraint equal A6 A7
  constraint coincident A6.start A7.end
  constraint coincident P3 L20
  constraint tangent L20 A8
  constraint tangent L19 A9
  constraint equal A8 A9
  constraint coincident A8.end A9.start
  measures "d130" distance of L9.start L9.end
  measures "d131" distance of L9.start P0
  measures "d132" distance of L9.start P1
  measures "d133" distance of L15.start L15.end
  measures "d134" distance of L15.start P2
  measures "d135" distance of L15.start P3
  measures "d136" radius of A2
  measures "d137" radius of A4
  measures "d138" radius of A6
  measures "d139" radius of A8
sketch "Sketch23" plane through (0, 75, 0) normal (0, 1, 0) x (-1, 0, 0)
  line L0 (-48.1, 13.6) -> (-48.1, 5.4)
  line L1 (-50.9, 5.4) -> (-50.9, 13.6)
  line L2 (-9.1, 13.6) -> (-9.1, 5.4)
  line L3 (-11.9, 5.4) -> (-11.9, 13.6)
  arc A0 (-10.5, 15) -> (-11.9, 13.6) centre (-10.5, 13.6) ccw
  arc A1 (-9.1, 13.6) -> (-10.5, 15) centre (-10.5, 13.6) ccw
  arc A2 (-11.9, 5.4) -> (-10.5, 4) centre (-10.5, 5.4) ccw
  arc A3 (-10.5, 4) -> (-9.1, 5.4) centre (-10.5, 5.4) ccw
  arc A4 (-49.5, 15) -> (-50.9, 13.6) centre (-49.5, 13.6) ccw
  arc A5 (-48.1, 13.6) -> (-49.5, 15) centre (-49.5, 13.6) ccw
  arc A6 (-50.9, 5.4) -> (-49.5, 4) centre (-49.5, 5.4) ccw
  arc A7 (-49.5, 4) -> (-48.1, 5.4) centre (-49.5, 5.4) ccw
  point P0 (-50.9, 15)
  point P1 (-48.1, 15)
  point P2 (-50.9, 4)
  point P3 (-11.9, 15)
  point P4 (-9.1, 15)
  point P5 (-11.9, 4)
  dimension "d140" = 2.8
  dimension "d141" = 11
  dimension "d142" = 2.8
  dimension "d143" = 11
  dimension "d144" = 1.4
  dimension "d145" = 1.4
  dimension "d146" = 1.4
  dimension "d147" = 1.4
  dimension "d148" = 1.4
  constraint vertical L0
  constraint vertical L1
  constraint vertical L2
  constraint vertical L3
  constraint coincident P3 L3
  constraint tangent L3 A0
  constraint coincident P4 L2
  constraint tangent L2 A1
  constraint coincident A0.start A1.end
  constraint coincident P5 L3
  constraint tangent L3 A2
  constraint tangent L2 A3
  constraint equal A2 A3
  constraint coincident A2.end A3.start
  constraint coincident P0 L1
  constraint tangent L1 A4
  constraint coincident P1 L0
  constraint tangent L0 A5
  constraint equal A4 A5
  constraint coincident A4.start A5.end
  constraint coincident P2 L1
  constraint tangent L1 A6
  constraint tangent L0 A7
  constraint equal A6 A7
  constraint coincident A6.end A7.start
  measures "d140" distance of P0 P1
  measures "d141" distance of P0 P2
  measures "d142" distance of P3 P4
  measures "d143" distance of P3 P5
  measures "d144" radius of A0
  measures "d145" radius of A1
  measures "d146" radius of A2
  measures "d147" radius of A4
  measures "d148" radius of A6
extrude "Extrude27" cut sketch "Sketch23" against normal blind 6
sketch "Sketch24" plane through (0, 70, 0) normal (0, -1, 0) x (1, 0, 0)
  line L0 (12.142, 10.8148) -> (13.733, 13.6294)
  line L1 (13.733, 13.6294) -> (12.091, 16.4146)
  line L2 (12.091, 16.4146) -> (8.858, 16.3852)
  line L3 (8.858, 16.3852) -> (7.267, 13.5706)
  line L4 (7.267, 13.5706) -> (8.909, 10.7854)
  line L5 (8.909, 10.7854) -> (12.142, 10.8148)
  line L6 (12.1166, 2.7) -> (13.7332, 5.5)
  line L7 (13.7332, 5.5) -> (12.1166, 8.3)
  line L8 (12.1166, 8.3) -> (8.8834, 8.3)
  line L9 (8.8834, 8.3) -> (7.2668, 5.5)
  line L10 (7.2668, 5.5) -> (8.8834, 2.7)
  line L11 (8.8834, 2.7) -> (12.1166, 2.7)
  line L12 (7.267, 13.5706) -> (7.2668, 5.5)
  line L13 (13.7332, 5.5) -> (13.733, 13.6294)
  line L14 (51.1166, 10.8) -> (52.7332, 13.6)
  line L15 (52.7332, 13.6) -> (51.1166, 16.4)
  line L16 (51.1166, 16.4) -> (47.8834, 16.4)
  line L17 (47.8834, 16.4) -> (46.2668, 13.6)
  line L18 (46.2668, 13.6) -> (47.8834, 10.8)
  line L19 (47.8834, 10.8) -> (51.1166, 10.8)
  line L20 (51.1203, 2.6022) -> (52.7332, 5.4043)
  line L21 (52.7332, 5.4043) -> (51.1128, 8.2022)
  line L22 (51.1128, 8.2022) -> (47.8797, 8.1978)
  line L23 (47.8797, 8.1978) -> (46.2668, 5.3957)
  line L24 (46.2668, 5.3957) -> (47.8872, 2.5978)
  line L25 (47.8872, 2.5978) -> (51.1203, 2.6022)
  line L26 (46.2668, 13.6) -> (46.2668, 5.3957)
  line L27 (52.7332, 5.4043) -> (52.7332, 13.6)
  point P0 (10.5, 13.6)
  point P1 (10.5, 5.5)
  point P2 (49.5, 13.6)
  point P3 (49.5, 5.4)
  dimension "d151" = 2.8
  dimension "d152" = 2.8
  dimension "d155" = 2.8
  dimension "d156" = 2.8
  measures "d151" distance of P0 L5
  measures "d152" distance of P1 L11
  measures "d155" distance of P2 L19
  measures "d156" distance of P3 L25
extrude "Extrude28" cut sketch "Sketch24" against normal blind 1.5 contours L0 L1 L2 L3 L4 L5 | L0 L4 L5 L7 L8 L9 L12 L13 | L6 L7 L8 L9 L10 L11
extrude "Extrude29" cut sketch "Sketch24" against normal blind 1.5 contours L14 L15 L16 L17 L18 L19 | L14 L18 L19 L21 L22 L23 L26 L27 | L20 L21 L22 L23 L24 L25
extrude "Extrude30" cut sketch "Sketch16" against normal blind 10 contours A1
sketch "Sketch25" plane through (60, 0, 0) normal (1, 0, 0) x (0, 1, 0)
  line L0 (42.5, 3) -> (42.5, 0)
  line L1 (42.5, 0) -> (72.5, 0)
  line L2 (72.5, 0) -> (72.5, 18)
  line L3 (72.5, 18) -> (2.5, 18)
  line L4 (2.5, 18) -> (2.5, 0)
  line L5 (2.5, 0) -> (32.5, 0)
  line L6 (32.5, 0) -> (32.5, 3)
  line L7 (32.5, 3) -> (42.5, 3)
  line L8 (31, 3) -> (44, 3)
  line L9 (44, 3) -> (44, 1.5)
  line L10 (44, 1.5) -> (31, 1.5)
  line L11 (31, 1.5) -> (31, 3)
  constraint horizontal L8
  constraint vertical L9
  constraint horizontal L10
  constraint vertical L11
extrude "Extrude31" cut sketch "Sketch25" against normal blind 55 contours L0 L8 L9 L10 | L0 L6 L7 L8 L10 | L6 L8 L10 L11
equation "d63 = 'USB PORT'"
equation "d65 = 'LED LAYER'"
